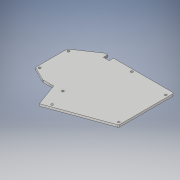
# Autodesk Inventor part: k2_base
Saved by Autodesk Inventor 2017 (Build 210142000, 142)
## iProperties
Created: 2017-02-07
Part Number: k2_base
Material: Generic
Document SubType Name: Modeling
Designer: herman
Density: 1 g/cm^3
Appearance: Default
Author: herman
Autodesk Inventor part; units mm, degrees
ref_plane "YZ Plane" through (0, 0, 0) normal (1, 0, 0) x (0, 1, 0)
ref_plane "XZ Plane" through (0, 0, 0) normal (0, 1, 0) x (-1, 0, 0)
ref_plane "XY Plane" through (0, 0, 0) normal (0, 0, 1) x (1, 0, 0)
sketch "Sketch8" plane through (0, 0, 0) normal (0, 1, 0) x (-1, 0, 0)
  line L0 (-67.0875, -125.7135) -> (28.9125, -125.7135)
  line L1 (24.9125, -50.7135) -> (13.6258, -19.7036)
  line L2 (39.9125, -50.7135) -> (24.9125, -50.7135)
  line L3 (-67.0875, -49.0809) -> (-67.0875, -125.7135)
  line L4 (13.6258, -19.7036) -> (-67.0875, -49.0809)
  line L5 (39.9125, -50.7135) -> (59.9125, -60.7135)
  line L6 (59.9125, -104.7135) -> (28.9125, -125.7135)
  line L7 (59.9125, -60.7135) -> (59.9125, -104.7135)
  dimension "d129" = 31
  dimension "d131" = 21
  dimension "d147" = 10
  dimension "d154" = 20
  dimension "d155" = 15
  dimension "d162" = 33
  dimension "d163" = 110
  dimension "d164" = 96
  dimension "d183" = 44
  constraints: 16 end point, 2 horizontal, 2 perpendicular, 1 vertical
  measures "d129" horizontal distance of L7.end L6.end
  measures "d131" vertical distance of L6.end L7.end
  measures "d147" vertical distance of L7.start L2.start
  measures "d154" horizontal distance of L7.start L2.start
  measures "d155" distance of L2.start L1.start
  measures "d162" distance of L1.start L1.end
  measures "d163" angle of L1 L2
  measures "d164" distance of L3.end L6.end
  measures "d183" distance of L7.start L7.end
extrude "Extrusion9" add sketch "Sketch8" along normal blind 3
sketch "Sketch9" plane through (0, 3, 0) normal (0, 1, 0) x (1, 0, 0)
  circle A0 centre (63.5875, 117.7135) radius 1.5
  circle A1 centre (-56.4125, 102.857) radius 1.5
  circle A2 centre (-56.4125, 62.8766) radius 1.5
  circle A3 centre (-3.7176, 27.5666) radius 1.5
  circle A4 centre (-12.2681, 51.059) radius 1.5
  line L0 (-24.9125, 50.7135) -> (-13.6258, 19.7036) projected
  line L1 (-13.6258, 19.7036) -> (67.0875, 49.0809) projected
  line L2 (67.0875, 49.0809) -> (67.0875, 125.7135) projected
  line L3 (67.0875, 125.7135) -> (-28.9125, 125.7135) projected
  line L4 (-28.9125, 125.7135) -> (-59.9125, 104.7135) projected
  line L5 (-59.9125, 104.7135) -> (-59.9125, 60.7135) projected
  line L6 (-59.9125, 60.7135) -> (-39.9125, 50.7135) projected
  line L7 (-39.9125, 50.7135) -> (-24.9125, 50.7135) projected
  line L8 (-56.4125, 102.857) -> (-27.8386, 122.2135) construction
  line L9 (-27.8386, 122.2135) -> (63.5875, 122.2135) construction
  line L10 (63.5875, 122.2135) -> (63.5875, 51.5316) construction
  line L11 (63.5875, 51.5316) -> (-11.534, 24.1896) construction
  line L12 (-11.534, 24.1896) -> (-22.4618, 54.2135) construction
  line L13 (-22.4618, 54.2135) -> (-39.0863, 54.2135) construction
  line L14 (-39.0863, 54.2135) -> (-56.4125, 62.8766) construction
  line L15 (-56.4125, 62.8766) -> (-56.4125, 102.857) construction
  line L16 (-39.9125, 50.7135) -> (-24.9125, 50.7135) construction
  line L17 (-24.9125, 50.7135) -> (-21.6236, 51.9106) construction
  circle A5 centre (63.5875, 52.5809) radius 1.5
  line L18 (-24.9125, 50.7135) -> (-13.6258, 19.7036) construction
  line L19 (-23.5444, 46.9547) -> (-12.2681, 51.059) construction
  circle A6 centre (12.0875, 122.2135) radius 1.5
  point P0 (0, 0)
  dimension "d135" = 3
  dimension "d136" = 3
  dimension "d137" = 3
  dimension "d165" = 3
  dimension "d166" = 3
  dimension "d169" = 3.5
  dimension "d185" = 3
  dimension "d186" = 3.5
  dimension "d187" = 3.5
  dimension "d191" = 12
  dimension "d193" = 4
  dimension "d194" = 12
  dimension "d195" = 4
  dimension "d204" = 8
  dimension "d205" = 3
  dimension "d206" = 55
  constraints: 20 end point, 7 centre point, 4 point on line, 3 coincident, 2 perpendicular, 7 other
  measures "d135" diameter of A2
  measures "d136" diameter of A1
  measures "d137" diameter of A0
  measures "d165" diameter of A3
  measures "d166" diameter of A4
  measures "d169" distance between parallel lines of L4 L8
  measures "d185" diameter of A5
  measures "d186" horizontal distance of L1.end A5.centre
  measures "d187" horizontal distance of A5.centre L1.end
  measures "d191" distance of L19.start L19.end
  measures "d193" distance between parallel lines of L17 L19
  measures "d194" distance from line of L0 A3.centre
  measures "d195" distance from line of L1 A3.centre
  measures "d204" distance from line of L3 A0.centre
  measures "d205" diameter of A6
  measures "d206" distance from line of L2 A6.centre
extrude "Extrusion10" cut sketch "Sketch9" against normal through all contours A0 | A1 | A2 | A3 | A4 | A5 | A6
sketch "Sketch10" plane through (0, 3, 0) normal (0, 1, 0) x (1, 0, 0)
  line L0 (-28.9125, 125.7135) -> (-59.9125, 104.7135) projected
  line L1 (67.0875, 125.7135) -> (-28.9125, 125.7135) projected
  line L2 (-24.9125, 125.7135) -> (-16.9125, 125.7135)
  line L3 (-16.9125, 125.7135) -> (-16.9125, 119.7135)
  line L4 (-16.9125, 119.7135) -> (-24.9125, 119.7135)
  line L5 (-24.9125, 119.7135) -> (-24.9125, 125.7135)
  point P0 (-17.0619, -65.3949)
  dimension "d179" = 4
  dimension "d180" = 6
  dimension "d181" = 8
  constraints: 8 end point, 2 parallel, 1 horizontal, 1 perpendicular, 1 point on line
  measures "d179" distance of L0.start L2.start
  measures "d180" distance of L4.end L2.start
  measures "d181" distance of L3.end L4.end
extrude "Extrusion11" cut sketch "Sketch10" against normal through all
fillet "Fillet1" radius 2 1 edges at (-39.9125, 1.5, -50.7135)
fillet "Fillet2" radius 2 1 edges at (-59.9125, 1.5, -60.7135)
fillet "Fillet3" radius 2 1 edges at (-59.9125, 1.5, -104.7135)
fillet "Fillet4" radius 2 1 edges at (-28.9125, 1.5, -125.7135)
fillet "Fillet5" radius 2 1 edges at (67.0875, 1.5, -125.7135)
fillet "Fillet6" radius 2 1 edges at (67.0875, 1.5, -49.0809)
body "Solid5"
